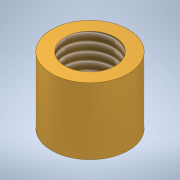
# Autodesk Inventor part: UD-43040
Saved by Autodesk Inventor 2022.3 (Build 263350000, 350)
## iProperties
Part Number: UD-43040
Material: 真鍮
Document SubType Name: Modeling
Designer: Masato Kubotera
Density: 5.62801 g/cm^3
Appearance: 真鍮 - サテン
Mass: 0.215 g
Surface Area: 1.14605 cm^2
Volume: 0.0382018 cm^3
Description: ReadyMade
Catalog Web Link: https://jp.misumi-ec.com/vona2/detail/221000748262/?HissuCode=UD-43040
Author: Masato Kubotera
Autodesk Inventor part; units mm, degrees
ref_plane "YZ Plane" through (0, 0, 0) normal (1, 0, 0) x (0, 1, 0)
ref_plane "XZ Plane" through (0, 0, 0) normal (0, 1, 0) x (-1, 0, 0)
ref_plane "XY Plane" through (0, 0, 0) normal (0, 0, 1) x (1, 0, 0)
sketch "スケッチ1" plane through (0, 0, 0) normal (0, 1, 0) x (-1, 0, 0)
  line L0 (0, 4) -> (0, 0) construction
  line L1 (1.5, 4) -> (1.5, 0)
  line L2 (1.5, 0) -> (2.3, 0)
  line L3 (2.3, 0) -> (2.3, 4)
  line L4 (2.3, 4) -> (1.5, 4)
  dimension "d1" = 4
  dimension "d6" = 3
  dimension "d7" = 4.6
  constraints: 10 end point, 3 perpendicular, 2 point on line, 2 vertical
  measures "d1" distance of L2.end L3.end
  measures "d6" diameter of L1 L0
  measures "d7" diameter of L3 L0
revolve "回転1" add sketch "スケッチ1" angle 360 about axis through (0, 0, 4) along (0, 0, -1)
thread "ねじ1" size "M3x0.5" class "6H" standard "ANSI Metric M Profile" full length
